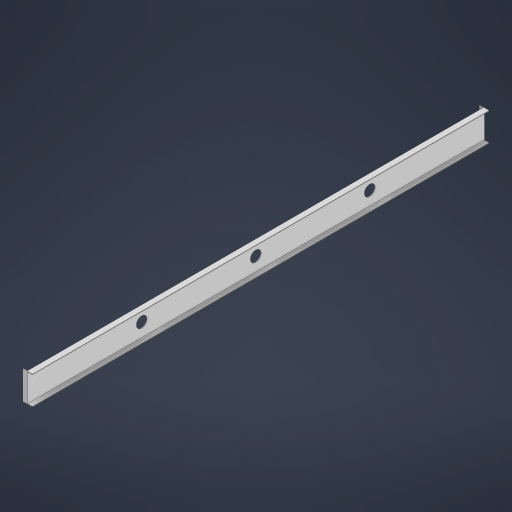
# Autodesk Inventor part: Chassis SideV1
Saved by Autodesk Inventor 2023 (Build 270158000, 158)
## iProperties
Created: 2022-04-13
Part Number: Chassis SideV1
Material: Generic
Document SubType Name: Modeling
Designer: timmy
Density: 1 g/cm^3
Appearance: Default
Author: timmy
Autodesk Inventor part; units mm, degrees
ref_plane "YZ Plane" through (0, 0, 0) normal (1, 0, 0) x (0, 1, 0)
ref_plane "XZ Plane" through (0, 0, 0) normal (0, 1, 0) x (-1, 0, 0)
ref_plane "XY Plane" through (0, 0, 0) normal (0, 0, 1) x (1, 0, 0)
sketch "Sketch1" plane through (0, 0, 0) normal (1, 0, 0) x (0, 1, 0)
  line L0 (0, 0) -> (76.2, 0)
  line L1 (76.2, 0) -> (76.2, -1219.2)
  line L2 (76.2, -1219.2) -> (0, -1219.2)
  line L3 (0, -1219.2) -> (0, 0)
  dimension "d0" = 76.2
  dimension "d1" = 1219.2
  constraints: 8 end point, 2 parallel, 1 horizontal, 1 perpendicular
  measures "d0" distance of L1.end L2.end
  measures "d1" distance of L0.end L1.end
extrude "Extrusion1" add sketch "Sketch1" along normal blind 1.5875
sketch "Sketch2" plane through (0, 0, 0) normal (0, 0, 1) x (1, 0, 0)
  line L0 (0, 76.2) -> (0, 0) projected
  line L1 (0, 0) -> (1.5875, 0) projected
  line L2 (1.5875, 76.2) -> (1.5875, 0) projected
  line L3 (0, 76.2) -> (1.5875, 76.2) projected
  line L4 (1.5875, 0) -> (-11.1125, 0)
  line L5 (-11.1125, 0) -> (-11.1125, 76.2)
  line L6 (-11.1125, 76.2) -> (1.5875, 76.2)
  line L7 (1.5875, 76.2) -> (1.5875, 0)
  dimension "d4" = 12.7
  constraints: 8 end point, 2 parallel, 1 horizontal, 1 perpendicular
  measures "d4" distance of L5.end L6.end
extrude "Extrusion2" add sketch "Sketch2" against normal blind 1.5875 contours L0 L4 L5 L6
sketch "Sketch3" plane through (0, 0, -1219.2) normal (0, 0, -1) x (-1, 0, 0)
  line L0 (0, 0) -> (11.1125, 0) projected
  line L1 (11.1125, 0) -> (11.1125, 76.2) projected
  line L2 (11.1125, 76.2) -> (0, 76.2) projected
  line L3 (0, 0) -> (0, 76.2) projected
extrude "Extrusion3" add sketch "Sketch3" against normal blind 1.5875
sketch "Sketch5" plane through (1.5875, 76.2, 0) normal (0, 1, 0) x (1, 0, 0)
  line L0 (-1.5875, 1217.6125) -> (-1.5875, 1.5875) projected
  line L1 (-12.7, 1.5875) -> (-1.5875, 1.5875) projected
  line L2 (-12.7, 0) -> (-12.7, 1.5875) projected
  line L3 (-12.7, 0) -> (0, 0) projected
  line L4 (0, 1219.2) -> (0, 0) projected
  line L5 (-12.7, 1219.2) -> (0, 1219.2) projected
  line L6 (-12.7, 1219.2) -> (-12.7, 1217.6125) projected
  line L7 (-1.5875, 1217.6125) -> (-12.7, 1217.6125) projected
  line L8 (0, 0) -> (12.7, 0)
  line L9 (12.7, 0) -> (12.7, 1219.2)
  line L10 (12.7, 1219.2) -> (0, 1219.2)
  line L11 (0, 1219.2) -> (0, 0)
  point P0 (-1.5875, 0)
  dimension "d13" = 12.7
  constraints: 8 end point, 2 parallel, 1 horizontal, 1 perpendicular
  measures "d13" distance of L10.end L9.end
extrude "Extrusion4" add sketch "Sketch5" against normal blind 1.5875 contours L10 L9 L8 L4
sketch "Sketch6" plane through (1.5875, 0, -1219.2) normal (0, -1, 0) x (1, 0, 0)
  line L0 (12.7, 0) -> (12.7, 1219.2) projected
  line L1 (12.7, 1219.2) -> (0, 1219.2) projected
  line L2 (0, 0) -> (0, 1219.2) projected
  line L3 (0, 0) -> (12.7, 0) projected
  point P0 (-1.5875, 1219.2)
extrude "Extrusion5" add sketch "Sketch6" against normal blind 1.5875
sketch "Sketch7" plane through (1.5875, 0, 0) normal (1, 0, 0) x (0, 0, -1)
  line L0 (0, 1.5875) -> (1219.2, 1.5875) projected
  line L1 (1219.2, 1.5875) -> (1219.2, 74.6125) projected
  line L2 (1219.2, 74.6125) -> (0, 74.6125) projected
  line L3 (0, 74.6125) -> (0, 1.5875) projected
  line L4 (0, 38.1) -> (1217.6125, 38.1)
  line L5 (1217.6125, 76.2) -> (1217.6125, 0) projected
  line L6 (608.8062, 38.1) -> (608.8062, 66.0202)
  line L7 (608.8062, 66.0202) -> (0, 66.0202)
  line L8 (304.4031, 66.0202) -> (304.4031, 38.1)
  circle A0 centre (304.4031, 38.1) radius 14.3002
  circle A1 centre (608.8062, 38.1) radius 14.3002
  circle A2 centre (913.2094, 38.1) radius 14.3002
  point P0 (0, 0)
  dimension "d18" = 28.6004
  dimension "d19" = 28.6004
  constraints: 8 end point, 4 midpoint, 3 centre point, 2 coincident, 2 perpendicular, 2 point on line, 1 symmetric about line, 1 vertical, 1 other
  measures "d18" diameter of A0
  measures "d19" diameter of A1
extrude "Extrusion6" cut sketch "Sketch7" against normal blind 25.4 contours A0 L8 L4 | L4 A0 | A2 L4 | L4 A2 | L8 A0 L4 | A1 L6 L4 | L4 A1 | L4 L6 A1
body "Solid1"
